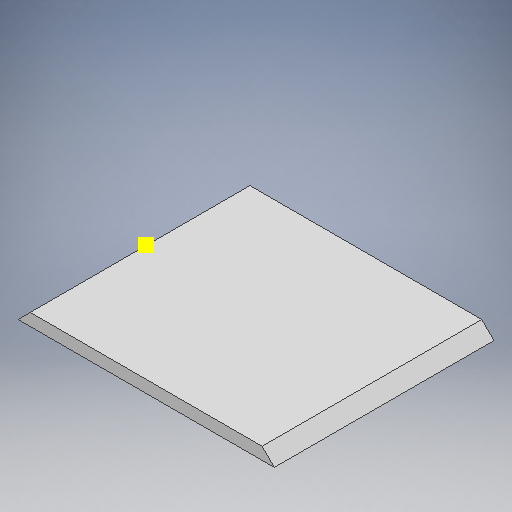
# Autodesk Inventor part: front_fender
Saved by Autodesk Inventor 2025.2 (Build 292293000, 293)
## iProperties
Created: 2025-02-07
Part Number: front_fender
Material: 일반
Document SubType Name: Modeling
Designer: jbhma
Density: 1 g/cm^3
Appearance: 기본값
Author: jbhma
Autodesk Inventor part; units mm, degrees
ref_plane "YZ Plane" through (0, 0, 0) normal (1, 0, 0) x (0, 1, 0)
ref_plane "XZ Plane" through (0, 0, 0) normal (0, 1, 0) x (-1, 0, 0)
ref_plane "XY Plane" through (0, 0, 0) normal (0, 0, 1) x (1, 0, 0)
sketch "스케치1" plane through (0, 0, 0) normal (0, 1, 0) x (-1, 0, 0)
  line L0 (-0.288, 0) -> (-420.288, 0)
  line L1 (-420.288, 0) -> (-420.288, -360)
  line L2 (-420.288, -360) -> (-0.288, -360)
  line L3 (-0.288, -360) -> (-0.288, 0)
  point P0 (0, 0)
  dimension "d0" = 420
  dimension "d1" = 360
  constraints: 8 end point, 2 parallel, 1 horizontal, 1 perpendicular
  measures "d0" distance of L2.end L1.end
  measures "d1" distance of L1.end L0.end
extrude "돌출1" add sketch "스케치1" along normal blind 20
chamfer "모따기1" distance 20 angle 45 1 edges at (420.288, 20, -180)
chamfer "모따기2" distance 20 angle 45 1 edges at (0.288, 20, -180)
sketch "스케치2" plane through (420.288, 0, -360) normal (0.7071068, 0.7071068, 0) x (-0.7071068, 0.7071068, 0)
  point P0 (297.1885, 360)
